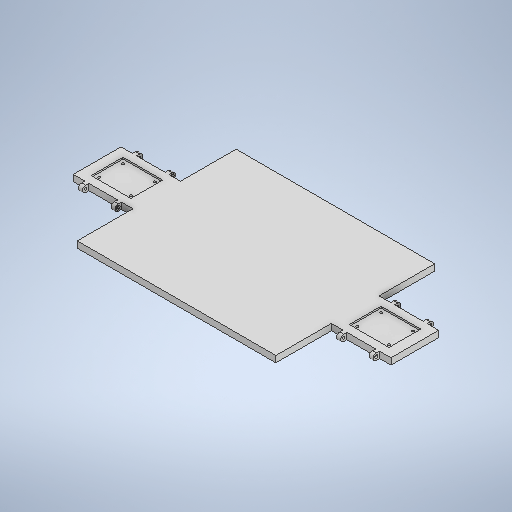
# Autodesk Inventor part: RC 하단프레임!
Saved by Autodesk Inventor 2025.2 (Build 292293000, 293)
## iProperties
Created: 2025-01-03
Part Number: RC 하단프레임!
Material: 일반
Document SubType Name: Modeling
Designer: kkk
Density: 1 g/cm^3
Appearance: 기본값
Author: kkk
Autodesk Inventor part; units mm, degrees
ref_plane "YZ Plane" through (0, 0, 0) normal (1, 0, 0) x (0, 1, 0)
ref_plane "XZ Plane" through (0, 0, 0) normal (0, 1, 0) x (-1, 0, 0)
ref_plane "XY Plane" through (0, 0, 0) normal (0, 0, 1) x (1, 0, 0)
sketch "스케치1" plane through (0, 0, 0) normal (0, 1, 0) x (-1, 0, 0)
  line L0 (-125, -100) -> (-125, -30)
  line L1 (-125, -30) -> (-200, -30)
  line L2 (125, -100) -> (125, -30)
  line L3 (125, -30) -> (200, -30)
  line L4 (-200, 0) -> (200, 0)
  line L5 (-125, 100) -> (-125, 30)
  line L6 (-125, 30) -> (-200, 30)
  line L7 (125, 100) -> (125, 30)
  line L8 (125, 30) -> (200, 30)
  line L9 (-200, -30) -> (-200, 30)
  line L10 (-125, 100) -> (125, 100)
  line L11 (200, 30) -> (200, -30)
  line L12 (-125, -100) -> (125, -100)
  line L13 (-125, 30) -> (-125, -30)
  line L14 (-142.5, -15) -> (-182.5, -15)
  line L15 (-182.5, -15) -> (-182.5, 15)
  line L16 (-182.5, 15) -> (-142.5, 15)
  line L17 (-142.5, 15) -> (-142.5, -15)
  line L18 (-142.5, -15) -> (-182.5, 15) construction
  line L19 (-182.5, -15) -> (-142.5, 15) construction
  point P0 (0, 0)
  point P1 (-162.5, 0)
  dimension "d13" = 70
  dimension "d14" = 75
  dimension "d15" = 70
  dimension "d16" = 75
  dimension "d17" = 250
  dimension "d18" = 60
  dimension "d19" = 40
  dimension "d20" = 30
  constraints: 40 end point, 6 symmetric about line, 5 horizontal, 4 coincident, 2 midpoint, 2 parallel, 2 perpendicular, 2 vertical, 1 collinear, 1 point on line, 1 other
  measures "d13" distance of L0.start L0.end
  measures "d14" distance of L0.end L1.end
  measures "d15" distance of L2.start L2.end
  measures "d16" distance of L2.end L3.end
  measures "d17" distance of L5.start L7.start
  measures "d18" distance between parallel lines of L6 L1
  measures "d19" distance of L15.end L16.end
  measures "d20" distance of L14.end L15.end
extrude "돌출1" add sketch "스케치1" along normal blind 8
hole "구멍1" at (182.5, 0, 15) at (142.5, 0, 15) at (142.5, 0, -15) at (182.5, 0, -15) direction (0, 1, 0) diameter 3 end through all counterbore diameter 4 counterbore depth 2
sketch "스케치2" plane through (0, 8, 0) normal (0, 1, 0) x (1, 0, 0)
  circle A0 centre (182.5, 15) radius 1.5 projected
  circle A1 centre (142.5, 15) radius 1.5 projected
  circle A2 centre (142.5, -15) radius 1.5 projected
  circle A3 centre (182.5, -15) radius 1.5 projected
  line L0 (200, -30) -> (200, 30) projected
  line L1 (200, 30) -> (125, 30) projected
  line L2 (125, 30) -> (125, 100) projected
  line L3 (125, 100) -> (-125, 100) projected
  line L4 (-125, 100) -> (-125, 30) projected
  line L5 (-125, 30) -> (-200, 30) projected
  line L6 (-200, 30) -> (-200, -30) projected
  line L7 (-200, -30) -> (-125, -30) projected
  line L8 (-125, -30) -> (-125, -100) projected
  line L9 (-125, -100) -> (125, -100) projected
  line L10 (125, -100) -> (125, -30) projected
  line L11 (125, -30) -> (200, -30) projected
  line L12 (137.5, 20) -> (187.5, 20)
  line L13 (187.5, 20) -> (187.5, -20)
  line L14 (187.5, -20) -> (137.5, -20)
  line L15 (137.5, -20) -> (137.5, 20)
  line L16 (137.5, 20) -> (187.5, -20) construction
  line L17 (187.5, 20) -> (137.5, -20) construction
  point P0 (0, 0)
  point P1 (162.5, 0)
  dimension "d30" = 50
  dimension "d31" = 40
  constraints: 12 end point, 2 midpoint, 2 parallel, 1 horizontal, 1 perpendicular, 1 other
  measures "d30" distance of L13.end L14.end
  measures "d31" distance of L12.end L13.end
extrude "돌출2" cut sketch "스케치2" against normal blind 2 contours L12 L13 L14 L15
sketch "스케치3" plane through (200, 0, -30) normal (0, 0, -1) x (-1, 0, 0)
  line L0 (75, 8) -> (0, 8) projected
  line L1 (37.5, 8) -> (0, 8)
  line L2 (75, 0) -> (0, 0) projected
  line L3 (75, 8) -> (325, 8) projected
  line L4 (75, 8) -> (37.5, 8)
  line L5 (14.5, 8) -> (19.5, 8)
  line L6 (19.5, 8) -> (19.5, 0)
  line L7 (19.5, 0) -> (14.5, 0)
  line L8 (14.5, 0) -> (14.5, 8)
  line L9 (14.5, 8) -> (19.5, 0) construction
  line L10 (19.5, 8) -> (14.5, 0) construction
  line L11 (55.5, 8) -> (60.5, 8)
  line L12 (60.5, 8) -> (60.5, 0)
  line L13 (60.5, 0) -> (55.5, 0)
  line L14 (55.5, 0) -> (55.5, 8)
  line L15 (55.5, 8) -> (60.5, 0) construction
  line L16 (60.5, 8) -> (55.5, 0) construction
  line L17 (62.5, 8) -> (12.5, 8) projected
  line L18 (0, 8) -> (75, 8) projected
  point P0 (200, 0)
  point P1 (17, 4)
  point P2 (58, 4)
  point P3 (60.5, 8)
  point P4 (55.5, 8)
  point P5 (55.5, 0)
  point P6 (14.5, 0)
  point P7 (37.5, 8)
  point P8 (37.5, 8)
  dimension "d34" = 5
  dimension "d35" = 5
  dimension "d49" = 36
  dimension "d51" = 18
  constraints: 28 end point, 6 midpoint, 4 parallel, 2 collinear, 2 horizontal, 2 perpendicular, 2 point on line, 2 other
  measures "d34" distance of L6.end L7.end
  measures "d35" distance of L12.end L13.end
  measures "d49" distance between parallel lines of L14 L6
  measures "d51" distance from line of L6 point (37.5, 8)
extrude "돌출3" add sketch "스케치3" along normal blind 8 contours L12 L2 L14 L0 | L6 L2 L8 L0
fillet "모깎기1" radius 4 4 edges at (183, 0, -38) (142, 0, -38) (142, 8, -38) (183, 8, -38)
sketch "스케치5" plane through (185.5, 0, -30) normal (1, 0, 0) x (0, 0, -1)
  arc A0 (4, 0) -> (4, 8) centre (4, 4) ccw projected
  point P0 (-30, 0)
  constraints: 1 coincident
hole "구멍2" at (185.5, 4, -34) direction (-1, 0, 0) diameter 3 depth 46 counterbore diameter 4 counterbore depth 2
sketch "스케치6" plane through (139.5, 0, -30) normal (-1, 0, 0) x (0, 0, 1)
  circle A0 centre (-4, 4) radius 1.5 projected
  line L0 (-1.25, 4) -> (-2.625, 1.6184)
  line L1 (-2.625, 1.6184) -> (-5.375, 1.6184)
  line L2 (-5.375, 1.6184) -> (-6.75, 4)
  line L3 (-6.75, 4) -> (-5.375, 6.3816)
  line L4 (-5.375, 6.3816) -> (-2.625, 6.3816)
  line L5 (-2.625, 6.3816) -> (-1.25, 4)
  point P0 (30, 0)
  dimension "d46" = 5.5
  constraints: 12 end point, 1 coincident, 13 other
  measures "d46" distance of L2.end L0.start
extrude "돌출4" cut sketch "스케치6" against normal blind 2.4
mirror "미러1" about plane through (0, 0, 0) normal (0, 0, 1) of "돌출3", "모깎기1", "구멍2", "돌출4"
mirror "미러2" about plane through (0, 0, 0) normal (1, 0, 0) of "돌출3", "모깎기1", "구멍2", "돌출4", "미러1"
mirror "미러3" about plane through (0, 0, 0) normal (1, 0, 0) of "구멍1", "돌출2"
equation "\"d51\" = 0.5 * d49"
